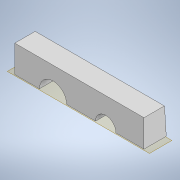
# Autodesk Inventor part: waterSoftenerDrainPipes
Saved by Autodesk Inventor 2021.1 (Build 251245000, 245)
## iProperties
Created: 2020-08-29
Part Number: waterSoftenerDrainPipes
Material: Generic
Document SubType Name: Modeling
Designer: robst
Density: 1 g/cm^3
Appearance: Default
Author: robst
Autodesk Inventor part; units mm, degrees
ref_plane "YZ Plane" through (0, 0, 0) normal (1, 0, 0) x (0, 1, 0)
ref_plane "XZ Plane" through (0, 0, 0) normal (0, 1, 0) x (-1, 0, 0)
ref_plane "XY Plane" through (0, 0, 0) normal (0, 0, 1) x (1, 0, 0)
sketch "Sketch1" plane through (0, 0, 0) normal (1, 0, 0) x (0, 1, 0)
  line L0 (0, 0) -> (0, 15.24)
  line L1 (0, 0) -> (-101.6, 0) construction
  arc A0 (-101.6, 0) -> (0, 0) centre (-50.8, 607.4796) ccw
  line L2 (-50.8, -2.1204) -> (-50.8, 0) construction
  line L3 (0, 15.24) -> (101.6, 15.24) construction
  arc A1 (0, 15.24) -> (101.6, 15.24) centre (50.8, 622.7196) ccw construction
  line L4 (-101.6, 0) -> (-101.6, 15.24)
  line L5 (-101.6, 15.24) -> (0, 15.24)
  dimension "d0" = 15.24
  dimension "d1" = 101.6
  dimension "d3" = 50.8
  dimension "d4" = 2.1204
  dimension "d5" = 609.6
  dimension "d6" = 101.6
  dimension "d7" = 609.6
  constraints: 12 end point, 5 point on circle, 2 centre point, 2 horizontal, 2 vertical, 1 midpoint, 1 parallel
  measures "d0" distance of L0.start L0.end
  measures "d1" distance of L0.start L1.end
  measures "d3" distance of L2.end L0.start
  measures "d4" distance of L2.start L2.end
  measures "d5" radius of A0
  measures "d6" distance of L0.end L3.end
  measures "d7" radius of A1
extrude "Extrusion1" add sketch "Sketch1" along normal mid plane 96.52
sketch "Sketch2" plane through (-48.26, -101.6, 15.24) normal (0, 0, 1) x (1, 0, 0)
  line L0 (48.26, 101.6) -> (48.26, 0) construction
  line L1 (0, 0) -> (96.52, 0) construction
  line L2 (0, 0) -> (0, 101.6) construction
  line L3 (0, 81.28) -> (96.52, 81.28) construction
  circle A0 centre (28.575, 81.28) radius 10.16
  circle A1 centre (67.945, 81.28) radius 7.62
  line L4 (0, 101.6) -> (96.52, 101.6) projected
  dimension "d11" = 20.32
  dimension "d12" = 15.24
  dimension "d13" = 57.15
  dimension "d14" = 19.685
  dimension "d20" = 20.32
  constraints: 4 end point, 3 point on line, 2 centre point, 1 horizontal, 1 midpoint
  measures "d11" diameter of A0
  measures "d12" diameter of A1
  measures "d14" distance from line of A0.centre L0
  measures "d20" distance between parallel lines of L3 L4
extrude "Extrusion2" cut sketch "Sketch2" against normal through all
ref_plane "Work Plane1" through (-48.26, -20.32, 15.24) normal (0, 1, 0) x (1, 0, 0)
split "Split1" plane through (-48.26, -20.32, 15.24) removes the side toward (0, -1, 0)
equation "\"d0\" = sidingDepth"
equation "\"d1\" = sidingHeight"
equation "\"d5\" = radiusOfCurvature"
equation "\"d6\" = sidingHeight"
equation "\"d7\" = radiusOfCurvature"
equation "\"d9\" = overallWidth"
equation "\"d11\" = leftPipeDiameter"
equation "\"d12\" = rightPipeDiameter"
equation "\"d13\" = outerDistanceBetweenPipep"
equation "\"d14\" = centerOfLeftPipe"
equation "\"d20\" = centerLineOfPipes"
equation "\"sidingHeight\" = 101.6"
equation "\"sidingDepth\" = 15.24"
equation "\"radiusOfCurvature\" = 609.6"
equation "\"centerLineOfPipes\" = 20.32"
equation "\"outerDistanceBetweenPipep\" = 57.15"
equation "\"leftPipeDiameter\" = 20.32"
equation "\"rightPipeDiameter\" = 15.24"
equation "\"overallWidth\" = 96.52"
equation "\"centerOfLeftPipe\" = 19.685"
equation "\"d21\" = -centerLineOfPipes"
body "Solid1"
